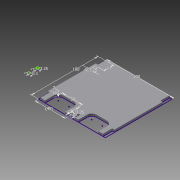
# Autodesk Inventor part: body-back
Saved by Autodesk Inventor 2013 (Build 170138000, 138)
## iProperties
Created: 2012-09-08
Part Number: body-back
Material: Generic
Document SubType Name: Modeling
Designer: frankenteddy
Density: 1 g/cm^3
Author: frankenteddy
Autodesk Inventor part; units mm, degrees
ref_plane "YZ Plane" through (0, 0, 0) normal (1, 0, 0) x (0, 1, 0)
ref_plane "XZ Plane" through (0, 0, 0) normal (0, 1, 0) x (-1, 0, 0)
ref_plane "XY Plane" through (0, 0, 0) normal (0, 0, 1) x (1, 0, 0)
sketch "Sketch1" plane through (0, 0, 0) normal (0, 0, 1) x (1, 0, 0)
  line L0 (-50, 50) -> (50, 50)
  line L1 (50, 50) -> (50, -50)
  line L2 (50, -50) -> (-50, -50)
  line L3 (-50, -50) -> (-50, 50)
  line L4 (-92.7646, -8.503) -> (-89.7646, -8.503)
  line L5 (-89.7646, -8.503) -> (-89.7646, -11.753)
  line L6 (-89.7646, -11.753) -> (-92.7646, -11.753)
  line L7 (-92.7646, -11.753) -> (-92.7646, -8.503)
  line L8 (-92.7646, -21.6527) -> (-89.7646, -21.6527)
  line L9 (-89.7646, -21.6527) -> (-89.7646, -21.7527)
  line L10 (-89.7646, -21.7527) -> (-92.7646, -21.7527)
  line L11 (-92.7646, -21.7527) -> (-92.7646, -21.6527)
  line L12 (-50, 50) -> (-46.75, 50)
  line L13 (-46.75, 50) -> (-46.75, 36)
  line L14 (-46.75, 36) -> (-50, 36)
  line L15 (-50, 36) -> (-50, 50)
  line L16 (0, 50) -> (0, -50) construction
  line L17 (-50, 0) -> (50, 0) construction
  line L18 (50, 50) -> (46.75, 50)
  line L19 (46.75, 50) -> (46.75, 36)
  line L20 (46.75, 36) -> (50, 36)
  line L21 (50, 36) -> (50, 50)
  line L22 (-50, -50) -> (-46.75, -50)
  line L23 (-46.75, -50) -> (-46.75, -36)
  line L24 (-46.75, -36) -> (-50, -36)
  line L25 (-50, -36) -> (-50, -50)
  line L26 (46.75, -50) -> (46.75, -36)
  line L27 (46.75, -36) -> (50, -36)
  line L28 (50, -36) -> (50, -50)
  line L29 (50, -50) -> (46.75, -50)
  line L30 (-40, -50) -> (-10, -50)
  line L31 (-10, -50) -> (-10, -37)
  line L32 (-17, -30) -> (-33, -30)
  line L33 (-40, -37) -> (-40, -50)
  line L34 (40, -50) -> (10, -50)
  line L35 (10, -50) -> (10, -37)
  line L36 (17, -30) -> (33, -30)
  line L37 (40, -37) -> (40, -50)
  line L38 (-1.75, -50) -> (-5, -50)
  line L39 (-5, -50) -> (-5, -42)
  line L40 (-5, -42) -> (-1.75, -42)
  line L41 (-1.75, -42) -> (-1.75, -50)
  line L42 (1.75, -50) -> (5, -50)
  line L43 (5, -50) -> (5, -42)
  line L44 (5, -42) -> (1.75, -42)
  line L45 (1.75, -42) -> (1.75, -50)
  arc A0 (-33, -30) -> (-40, -37) centre (-33, -37) ccw
  arc A1 (-10, -37) -> (-17, -30) centre (-17, -37) ccw
  arc A2 (17, -30) -> (10, -37) centre (17, -37) ccw
  arc A3 (40, -37) -> (33, -30) centre (33, -37) ccw
  point P0 (0, 0)
  point P1 (-10, -30)
  point P2 (-40, -30)
  point P3 (10, -30)
  point P4 (40, -30)
  dimension "d0" = 100
  dimension "d2" = 100
  dimension "d3" = 3
  dimension "mat" = 3.25
  dimension "d5" = 3
  dimension "kerf" = 0.1
  dimension "d7" = 3.25
  dimension "d8" = 14
  dimension "d15" = 30
  dimension "d16" = 20
  dimension "d17" = 10
  dimension "d20" = 3.25
  dimension "d21" = 8
  dimension "d22" = 5
  dimension "d25" = 45
  dimension "d26" = 7
  constraints: 92 end point, 17 symmetric about line, 12 parallel, 9 point on line, 8 point on circle, 8 tangent, 6 horizontal, 6 midpoint, 6 perpendicular, 4 centre point, 3 equal radius, 1 collinear
  measures "d0" distance of L0.start L0.end
  measures "d2" distance of L2.end L0.start
  measures "d3" distance of L5.end L6.end
  measures "mat" distance of L4.end L5.end
  measures "d5" distance of L9.end L10.end
  measures "kerf" distance of L8.end L9.end
  measures "d7" distance of L13.end L14.end
  measures "d8" distance of L12.end L13.end
  measures "d15" distance of point (-40, -30) point (-10, -30)
  measures "d16" distance of point (-10, -30) L30.end
  measures "d17" distance between parallel lines of L3 L33
  measures "d20" distance of L39.end L40.end
  measures "d21" distance of L38.end L39.end
  measures "d22" distance between parallel lines of L39 L31
  measures "d25" distance between parallel lines of L3 L39
  measures "d26" radius of A0
extrude "Extrusion2" add sketch "Sketch1" along normal blind 3.25 contours L0 L19 L20 L1 L27 L26 L2 L37 A3 L36 A2 L35 L43 L44 L45 L41 L40 L39 L31 A1 L32 A0 L33 L23 L24 L3 L14 L13 | L39 L40 L41 L2 | L45 L44 L43 L2
extrude "Extrusion3" cut sketch "Sketch1" along normal blind 3.25 contours L39 L40 L41 L2 | L45 L44 L43 L2
equation "\"d7\" = mat"
equation "\"d20\" = mat"
equation "\"d18\" = mat"
equation "\"d23\" = mat"
body "Solid2"
